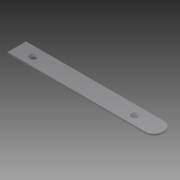
# Autodesk Inventor part: 13_1087_041
Saved by Autodesk Inventor 2014 SP1 (Build 180222100, 222)
## iProperties
Created: 2013-09-20
Part Number: 13_1087_041
Material: Allgemein
Document SubType Name: Modeling
Designer: vogel
Density: 1 g/cm^3
Appearance: Polycarbonat - klar
Author: vogel
Autodesk Inventor part; units mm, degrees
ref_plane "YZ Plane" through (0, 0, 0) normal (1, 0, 0) x (0, 1, 0)
ref_plane "XZ Plane" through (0, 0, 0) normal (0, 1, 0) x (-1, 0, 0)
ref_plane "XY Plane" through (0, 0, 0) normal (0, 0, 1) x (1, 0, 0)
sketch "Skizze1" plane through (0, 0, 0) normal (0, 0, 1) x (1, 0, 0)
  line L0 (-56, 0) -> (56, 0) projected
  line L1 (0, -7.7) -> (0, 7.7) projected
  line L2 (-40, 5.5) -> (40, 5.5)
  line L3 (40, 5.5) -> (40, -5.5)
  line L4 (40, -5.5) -> (-40, -5.5)
  line L5 (-40, -5.5) -> (-40, 5.5)
  point P0 (0, 0)
  dimension "d0" = 11
  dimension "d1" = 80
  constraints: 8 end point, 2 parallel, 1 horizontal, 1 perpendicular, 2 other
  measures "d0" distance of L2.end L3.end
  measures "d1" distance of L2.start L2.end
extrude "Extrusion1" add sketch "Skizze1" along normal blind 1
sketch "Skizze2" plane through (0, 0, 1) normal (0, 0, 1) x (1, 0, 0)
  line L0 (-140, 0) -> (140, 0) projected
  line L1 (0, -7.7) -> (0, 7.7) projected
  point P0 (0, 0)
  point P1 (-30, 0)
  point P2 (30, 0)
  dimension "d4" = 60
  constraints: 2 point on line, 1 symmetric about line
  measures "d4" distance of point (30, 0) point (-30, 0)
hole "Bohrung1" at (-30, 0, 1) at (30, 0, 1) direction (0, 0, -1) diameter 2.4 end through all countersink diameter 4.5 countersink angle 90
sketch "Skizze3" plane through (40, -5.5, 0) normal (1, 0, 0) x (0, 0, -1)
  line L0 (0, 11) -> (0, 0) projected
  line L1 (0, 11) -> (-1, 11) projected
  line L2 (-1, 0) -> (-1, 11) projected
  line L3 (0, 0) -> (-1, 0) projected
  point P0 (0, 5.5)
extrude "Extrusion2" add sketch "Skizze3" along normal blind 6.5
fillet "Rundung1" radius 5 2 edges at (46.5, -5.5, 0.5) (46.5, 5.5, 0.5)
